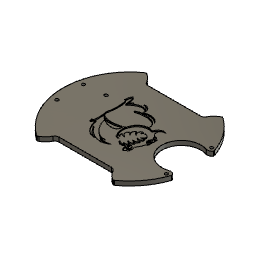
_lid.a9927ef6-e9e8-42fb-b627-377640e20614 (Autodesk Fusion 360 design; units mm, degrees)
Autodesk Fusion 360 part; units mm, degrees
sketch "reference" plane through (0, 0, 0) normal (0, 1, 0) x (1, 0, 0)
  line L0 (26.708, 42.6236) -> (27.1586, 42.6236)
  line L1 (-27.225, -55.0823) -> (17.225, -55.0823)
  line L2 (17.225, -55.0823) -> (17.225, -42.3823)
  line L3 (17.225, -42.3823) -> (-27.225, -42.3823)
  line L4 (-27.225, -42.3823) -> (-27.225, -55.0823)
  circle A0 centre (0, 0) radius 65
  line L5 (-27.225, 55.0823) -> (17.225, 55.0823)
  line L6 (17.225, 55.0823) -> (17.225, 42.3823)
  line L7 (17.225, 42.3823) -> (-27.225, 42.3823)
  line L8 (-27.225, 55.0823) -> (-27.225, 42.3823)
  circle A1 centre (0, 0) radius 67.15
  circle A2 centre (68.0978, 18.2467) radius 3
  circle A3 centre (68.0978, 18.2467) radius 1.425
  line L9 (0, 0) -> (82, 0) construction
  line L10 (0, 0) -> (-41, 71.0141) construction
  line L11 (0, 0) -> (-41, -71.0141) construction
  line L12 (87.4769, -0.0257) -> (79.614, 0.0081)
  line L13 (-39.814, 68.9437) -> (-43.7162, 75.77)
  line L14 (-39.8, -68.9518) -> (-43.7607, -75.7444)
  line L15 (0, 0) -> (70.5, 0) construction
  arc A4 (79.614, 0.0081) -> (74.6944, -3.9877) centre (79.5926, -4.9919) ccw
  arc A5 (-39.814, 68.9437) -> (-33.8938, 66.6811) centre (-35.4732, 71.4251) ccw
  arc A6 (-39.8, -68.9518) -> (-40.8007, -62.6934) centre (-44.1194, -66.4332) ccw
  spline S0 degree 5 poles (-33.8938, 66.6811) (-33.483, 66.8179) (-33.0729, 66.9532) (-32.6634, 67.087) (-32.2547, 67.2193) (-31.8466, 67.3502) knots 0.021144 0.021144 0.021144 0.021144 0.021144 0.021144 0.032444 0.032444 0.032444 0.032444 0.032444 0.032444
  line L16 (-32.0549, 67.2834) -> (-31.6382, 67.417)
  spline S1 degree 5 poles (5.0849, 74.3263) (6.6179, 74.3731) (11.2429, 74.4207) (18.7539, 74.0099) (28.746, 72.2391) (40.5731, 67.6689) (52.3904, 59.5578) (62.916, 48.5693) (72.252, 34.9305) (78.8493, 22.0782) (83.3385, 11.4171) (86.1309, 3.8631) (87.4769, -0.0257) knots 0.251095 0.251095 0.251095 0.251095 0.251095 0.251095 0.3 0.4 0.5 0.6 0.7 0.8 0.9 1 1 1 1 1 1
  line L17 (-9.3123, 73.8863) -> (19.482, 74.7663)
  spline S2 degree 5 poles (-40.8007, -62.6934) (-41.1245, -62.4061) (-41.4467, -62.1186) (-41.7673, -61.8309) (-42.0863, -61.543) (-42.4037, -61.255) knots 0.021144 0.021144 0.021144 0.021144 0.021144 0.021144 0.032444 0.032444 0.032444 0.032444 0.032444 0.032444
  line L18 (-42.2416, -61.4021) -> (-42.5658, -61.1079)
  spline S3 degree 5 poles (-66.9109, -32.7595) (-67.718, -31.4553) (-70.0717, -27.4737) (-73.4714, -20.7636) (-76.9339, -11.2248) (-78.8895, 1.3029) (-77.7737, 15.5925) (-73.5202, 30.2022) (-66.3767, 45.1068) (-58.5449, 57.2464) (-51.5568, 66.4647) (-46.4109, 72.66) (-43.7162, 75.77) knots 0.251095 0.251095 0.251095 0.251095 0.251095 0.251095 0.3 0.4 0.5 0.6 0.7 0.8 0.9 1 1 1 1 1 1
  line L19 (-59.9171, -44.0611) -> (-73.9047, -21.4578)
  arc A7 (-66.9109, -32.7595) -> (-37.25, -64.5189) centre (0, 0) ccw
  spline S4 degree 5 poles (74.6944, -3.9877) (74.6075, -4.4118) (74.5196, -4.8346) (74.4308, -5.2561) (74.341, -5.6763) (74.2503, -6.0951) knots 0.021144 0.021144 0.021144 0.021144 0.021144 0.021144 0.032444 0.032444 0.032444 0.032444 0.032444 0.032444
  line L20 (74.2965, -5.8814) -> (74.204, -6.3089)
  spline S5 degree 5 poles (61.826, -41.5668) (61.1001, -42.9178) (58.8287, -46.947) (54.7175, -53.2463) (48.1879, -61.0143) (38.3164, -68.9717) (25.3834, -75.1503) (10.6042, -78.7715) (-5.8753, -80.0373) (-20.3044, -79.3246) (-31.7817, -77.8819) (-39.7199, -76.523) (-43.7607, -75.7444) knots 0.251095 0.251095 0.251095 0.251095 0.251095 0.251095 0.3 0.4 0.5 0.6 0.7 0.8 0.9 1 1 1 1 1 1
  line L21 (68.2252, -29.657) -> (55.4268, -53.4766)
  arc A8 (61.826, -41.5668) -> (74.5, 0) centre (0, 0) ccw
  arc A9 (5.0849, 74.3263) -> (-37.25, 64.5189) centre (0, 0) ccw
  circle A10 centre (18.2467, 68.0978) radius 3
  circle A11 centre (18.2467, 68.0978) radius 1.425
  circle A12 centre (-49.851, 49.851) radius 3
  circle A13 centre (-49.851, 49.851) radius 1.425
  circle A14 centre (-68.0978, -18.2467) radius 3
  circle A15 centre (-68.0978, -18.2467) radius 1.425
  circle A16 centre (-18.2467, -68.0978) radius 3
  circle A17 centre (-18.2467, -68.0978) radius 1.425
  circle A18 centre (49.851, -49.851) radius 3
  circle A19 centre (49.851, -49.851) radius 1.425
  line L22 (0, 0) -> (55.15, 0) construction
  line L23 (0, 0) -> (55.15, 0) construction
  circle A20 centre (42.2474, -35.4497) radius 12
  circle A21 centre (42.2474, 35.4497) radius 12
  line L24 (0, 0) -> (55.15, 0) construction
  line L25 (0, 0) -> (55.15, 0) construction
  circle A22 centre (-42.2474, 35.4497) radius 12
  circle A23 centre (-42.2474, -35.4497) radius 12
  circle A24 centre (0, 0) radius 62.5
  line L26 (-5, -42.3823) -> (-5, 42.3823)
  point P0 (39, 67.55)
  point P1 (-78, 0)
  point P2 (39, -67.55)
  dimension "d9" = 12.7
  dimension "d10" = 44.45
  dimension "d53" = 12.7
  dimension "d54" = 44.45
  dimension "d63" = 130
  dimension "d76" = 134.3
  dimension "d123" = 78
  dimension "d127" = 5
  dimension "d128" = 5
  dimension "d129" = 5
  dimension "d132" = 149
  dimension "d136" = 360
  dimension "d204" = 55.15
  dimension "d206" = 55.15
  dimension "d207" = 24
  dimension "d208" = 24
  dimension "d210" = 55.15
  dimension "d212" = 55.15
  dimension "d213" = 24
  dimension "d214" = 24
  dimension "d227" = 125
  dimension "d232" = 84.7646
  constraint perpendicular L1 L2
  constraint perpendicular L2 L3
  constraint coincident A0.centre A1.centre
  constraint perpendicular L5 L6
  constraint perpendicular L6 L7
  constraint horizontal L9
  constraint horizontal L15
  constraint tangent A4 S4
  constraint tangent L12 A4
  constraint tangent A5 S0
  constraint tangent L13 A5
  constraint tangent A6 S2
  constraint tangent L14 A6
  constraint coincident S0.end A7
  constraint midpoint S0.end L16
  constraint coincident S1.start A7
  constraint midpoint S1.start L17
  constraint coincident L10 A9.end
  constraint coincident S2.end A7
  constraint midpoint S2.end L18
  constraint midpoint S3.start L19
  constraint coincident L11 A7.end
  constraint concentric A7 A8
  constraint coincident S4.end A8
  constraint midpoint S4.end L20
  constraint midpoint S5.start L21
  constraint coincident L9 A8.end
  constraint concentric A8 A9
  constraint horizontal L22
  constraint horizontal L23
  constraint horizontal L24
  constraint horizontal L25
  constraint midpoint L3 L26.start
  constraint midpoint L7 L26.end
  constraint perpendicular L7 L26
  measures "d9" distance of L1.end L2.end
  measures "d10" distance of L2.end L3.end
  measures "d53" distance of L5.end L6.end
  measures "d54" distance of L6.end L7.end
  measures "d63" diameter of A0
  measures "d76" diameter of A1
  measures "d123" distance of A0.centre P0
  measures "d127" radius of A4
  measures "d128" radius of A5
  measures "d129" radius of A6
  measures "d132" diameter of A7
  measures "d204" distance of A0.centre A20.centre
  measures "d206" distance of A0.centre A21.centre
  measures "d207" diameter of A20
  measures "d208" diameter of A21
  measures "d210" distance of A0.centre A23.centre
  measures "d212" distance of A0.centre A22.centre
  measures "d213" diameter of A22
  measures "d214" diameter of A23
  measures "d227" diameter of A24
  measures "d232" distance of L26.start L26.end
sketch "Sketch6" plane through (0, 0, 0) normal (0, 1, 0) x (1, 0, 0)
  line L0 (-18.5, 40.9998) -> (8.5, 40.9998)
  line L1 (24.1077, -40.9998) -> (-24.1077, -40.9998)
  line L2 (-18.5, 40.9998) -> (8.5, 40.9998)
  line L3 (-5, 40.9998) -> (-24.1077, 40.9998)
  line L4 (-5, 40.9998) -> (24.173, 40.9998)
  arc A0 (33.8961, 49.6132) -> (27.7096, 43.1311) centre (42.2474, 35.4497) ccw
  arc A1 (-27.6472, 43.1364) -> (-33.8408, 49.6476) centre (-42.2474, 35.4497) ccw
  arc A2 (-33.8408, -49.6476) -> (-27.6472, -43.1364) centre (-42.2474, -35.4497) ccw
  arc A3 (27.6472, -43.1364) -> (33.8408, -49.6476) centre (42.2474, -35.4497) ccw
  arc A4 (-24.1077, -40.9998) -> (-27.6472, -43.1364) centre (-24.1077, -44.9998) ccw
  arc A5 (27.6472, -43.1364) -> (24.1077, -40.9998) centre (24.1077, -44.9998) ccw
  arc A6 (24.173, 40.9998) -> (27.7096, 43.1311) centre (24.173, 44.9998) ccw
  arc A7 (-27.6472, 43.1364) -> (-24.1077, 40.9998) centre (-24.1077, 44.9998) ccw
  arc A8 (-33.8408, 49.6476) -> (-35.0849, 50.1261) centre (-35.8787, 46.2057) ccw
  arc A9 (35.1381, 50.0889) -> (33.8961, 49.6132) centre (35.9277, 46.1676) ccw
  arc A10 (-35.5399, -50.1913) -> (-33.8408, -49.6476) centre (-35.8787, -46.2057) ccw
  arc A11 (33.8408, -49.6476) -> (35.5399, -50.1913) centre (35.8787, -46.2057) ccw
  arc A12 (58.1788, -18.9422) -> (53.3811, -17.0548) centre (54.6603, -20.8448) ccw
  arc A13 (53.3811, 17.0548) -> (58.1788, 18.9422) centre (54.6603, 20.8448) ccw
  line L5 (25.625, -0.0248) -> (25.625, 0.0248)
  line L6 (-24.375, 0.0248) -> (-24.375, 0)
  line L7 (0, 0) -> (-24.375, 0) construction
  line L8 (-62.5, 0) -> (-63.5, 0) construction
  circle A14 centre (54.6603, 20.8448) radius 1.425
  circle A15 centre (54.6603, -20.8448) radius 1.425
  circle A16 centre (-54.8646, 12.1784) radius 1.425
  circle A17 centre (-54.8646, -12.1784) radius 1.425
  arc A18 (53.3811, 17.0548) -> (53.3811, -17.0548) centre (47.625, 0) ccw
  spline S0 degree 3 poles (23.6109, 1.2589) (23.5474, 1.4494) (23.3887, 1.7272) (23.2458, 1.8701) knots 0 0 0 0 1 1 1 1
  spline S1 degree 3 poles (23.2458, 1.8701) (22.6664, 2.4654) (21.9123, 2.2591) (21.0868, 1.2669) knots 0 0 0 0 1 1 1 1
  line L9 (21.0868, 1.2669) -> (20.8646, 1.0049)
  line L10 (20.8646, 1.0049) -> (20.6503, 1.2034)
  spline S2 degree 3 poles (20.6503, 1.2034) (20.5312, 1.3066) (20.3407, 1.4574) (20.2296, 1.5288) knots 0 0 0 0 1 1 1 1
  spline S3 degree 3 poles (20.2296, 1.5288) (20.0311, 1.6479) (19.6263, 2.1956) (19.6898, 2.2511) knots 0 0 0 0 1 1 1 1
  spline S4 degree 3 poles (19.6898, 2.2511) (19.7057, 2.2591) (19.8803, 2.3543) (20.0788, 2.4496) knots 0 0 0 0 1 1 1 1
  spline S5 degree 3 poles (20.0788, 2.4496) (20.4756, 2.648) (21.4281, 3.2671) (21.4281, 3.3306) knots 0 0 0 0 1 1 1 1
  spline S6 degree 3 poles (21.4281, 3.3306) (21.4281, 3.3544) (21.2614, 3.3624) (21.0551, 3.3465) knots 0 0 0 0 1 1 1 1
  spline S7 degree 3 poles (21.0551, 3.3465) (20.5391, 3.3068) (19.6739, 3.5211) (19.1183, 3.8148) knots 0 0 0 0 1 1 1 1
  spline S8 degree 3 poles (19.1183, 3.8148) (18.269, 4.2752) (17.5149, 5.2436) (17.253, 6.2278) knots 0 0 0 0 1 1 1 1
  spline S9 degree 3 poles (17.253, 6.2278) (17.1101, 6.7596) (17.1181, 7.6327) (17.2609, 8.2122) knots 0 0 0 0 1 1 1 1
  spline S10 degree 3 poles (17.2609, 8.2122) (17.6419, 9.6727) (18.8961, 10.8395) (20.428, 11.1649) knots 0 0 0 0 1 1 1 1
  spline S11 degree 3 poles (20.428, 11.1649) (20.7614, 11.2364) (21.1662, 11.2602) (21.4281, 11.2364) knots 0 0 0 0 1 1 1 1
  line L11 (21.4281, 11.2364) -> (21.8647, 11.1887)
  line L12 (21.8647, 11.1887) -> (21.571, 11.3475)
  spline S12 degree 3 poles (21.571, 11.3475) (20.6503, 11.8396) (19.0945, 11.8793) (17.9674, 11.4348) knots 0 0 0 0 1 1 1 1
  spline S13 degree 3 poles (17.9674, 11.4348) (16.4116, 10.8316) (15.2289, 9.7203) (14.4908, 8.1804) knots 0 0 0 0 1 1 1 1
  spline S14 degree 3 poles (14.4908, 8.1804) (14.3399, 7.855) (14.1733, 7.4105) (14.1177, 7.1803) knots 0 0 0 0 1 1 1 1
  line L13 (14.1177, 7.1803) -> (14.0224, 6.7596)
  line L14 (14.0224, 6.7596) -> (13.5779, 6.9104)
  spline S15 degree 3 poles (13.5779, 6.9104) (12.1492, 7.4026) (9.9743, 7.5613) (8.4424, 7.2756) knots 0 0 0 0 1 1 1 1
  spline S16 degree 3 poles (8.4424, 7.2756) (1.8146, 6.0532) (-2.5511, -1.1223) (-1.0191, -8.2581) knots 0 0 0 0 1 1 1 1
  spline S17 degree 3 poles (-1.0191, -8.2581) (-0.7334, -9.5996) (-0.1619, -11.1394) (0.6398, -12.7666) knots 0 0 0 0 1 1 1 1
  spline S18 degree 3 poles (0.6398, -12.7666) (1.1478, -13.7826) (2.1638, -14.5288) (3.1401, -14.5923) knots 0 0 0 0 1 1 1 1
  spline S19 degree 3 poles (3.1401, -14.5923) (3.6402, -14.624) (4.1244, -14.5208) (4.2672, -14.3462) knots 0 0 0 0 1 1 1 1
  spline S20 degree 3 poles (4.2672, -14.3462) (4.3307, -14.2748) (4.2593, -14.2509) (4.0132, -14.243) knots 0 0 0 0 1 1 1 1
  spline S21 degree 3 poles (4.0132, -14.243) (2.7591, -14.2113) (1.5129, -12.8936) (1.3224, -11.4173) knots 0 0 0 0 1 1 1 1
  spline S22 degree 3 poles (1.3224, -11.4173) (1.2907, -11.1871) (1.2986, -11.0363) (1.3462, -11.0363) knots 0 0 0 0 1 1 1 1
  spline S23 degree 3 poles (1.3462, -11.0363) (1.3939, -11.0363) (1.4256, -11.0839) (1.4256, -11.1474) knots 0 0 0 0 1 1 1 1
  spline S24 degree 3 poles (1.4256, -11.1474) (1.4256, -11.2109) (1.6082, -11.4569) (1.8225, -11.703) knots 0 0 0 0 1 1 1 1
  spline S25 degree 3 poles (1.8225, -11.703) (2.2194, -12.1316) (2.5686, -12.3221) (3.156, -12.4174) knots 0 0 0 0 1 1 1 1
  spline S26 degree 3 poles (3.156, -12.4174) (3.4259, -12.465) (3.5132, -12.3459) (3.2592, -12.2666) knots 0 0 0 0 1 1 1 1
  spline S27 degree 3 poles (3.2592, -12.2666) (3.0211, -12.1951) (2.4654, -11.5443) (2.2987, -11.1553) knots 0 0 0 0 1 1 1 1
  spline S28 degree 3 poles (2.2987, -11.1553) (2.0765, -10.6473) (1.9654, -9.8933) (2.0289, -9.4011) knots 0 0 0 0 1 1 1 1
  line L15 (2.0289, -9.4011) -> (2.0765, -8.9646)
  line L16 (2.0765, -8.9646) -> (2.3464, -9.2821)
  spline S29 degree 3 poles (2.3464, -9.2821) (2.9972, -10.0441) (4.1482, -10.56) (5.188, -10.56) knots 0 0 0 0 1 1 1 1
  spline S30 degree 3 poles (5.188, -10.56) (5.8468, -10.56) (6.1246, -10.4489) (5.6563, -10.3774) knots 0 0 0 0 1 1 1 1
  spline S31 degree 3 poles (5.6563, -10.3774) (4.8546, -10.2504) (3.7513, -9.3932) (3.3386, -8.5915) knots 0 0 0 0 1 1 1 1
  spline S32 degree 3 poles (3.3386, -8.5915) (2.5845, -7.1231) (2.9972, -5.5356) (4.299, -4.8926) knots 0 0 0 0 1 1 1 1
  line L17 (4.299, -4.8926) -> (4.7038, -4.6863)
  line L18 (4.7038, -4.6863) -> (4.9578, -5.0673)
  spline S33 degree 3 poles (4.9578, -5.0673) (5.2991, -5.5673) (5.8468, -6.0594) (6.3389, -6.3055) knots 0 0 0 0 1 1 1 1
  spline S34 degree 3 poles (6.3389, -6.3055) (6.5612, -6.4166) (6.7596, -6.5119) (6.7914, -6.5119) knots 0 0 0 0 1 1 1 1
  spline S35 degree 3 poles (6.7914, -6.5119) (6.8231, -6.5119) (6.6803, -6.3373) (6.4818, -6.1229) knots 0 0 0 0 1 1 1 1
  spline S36 degree 3 poles (6.4818, -6.1229) (5.1483, -4.7021) (5.2674, -2.4082) (6.7358, -1.2969) knots 0 0 0 0 1 1 1 1
  spline S37 degree 3 poles (6.7358, -1.2969) (6.9184, -1.1541) (7.1168, -1.035) (7.1803, -1.035) knots 0 0 0 0 1 1 1 1
  spline S38 degree 3 poles (7.1803, -1.035) (7.2359, -1.035) (7.3232, -1.2017) (7.3708, -1.4001) knots 0 0 0 0 1 1 1 1
  spline S39 degree 3 poles (7.3708, -1.4001) (7.6566, -2.5352) (8.6964, -3.6226) (9.7203, -3.8608) knots 0 0 0 0 1 1 1 1
  spline S40 degree 3 poles (9.7203, -3.8608) (9.9584, -3.9163) (9.9584, -3.9084) (9.6251, -3.6226) knots 0 0 0 0 1 1 1 1
  spline S41 degree 3 poles (9.6251, -3.6226) (8.5932, -2.7257) (8.2122, -1.1541) (8.744, 0.0048) knots 0 0 0 0 1 1 1 1
  spline S42 degree 3 poles (8.744, 0.0048) (9.1726, 0.9335) (9.7918, 1.3462) (10.7601, 1.3462) knots 0 0 0 0 1 1 1 1
  spline S43 degree 3 poles (10.7601, 1.3462) (11.0776, 1.3462) (11.3634, 1.3066) (11.3872, 1.2669) knots 0 0 0 0 1 1 1 1
  spline S44 degree 3 poles (11.3872, 1.2669) (11.411, 1.2192) (11.3634, 1.0764) (11.2681, 0.9494) knots 0 0 0 0 1 1 1 1
  spline S45 degree 3 poles (11.2681, 0.9494) (11.0538, 0.6477) (10.7919, -0.0904) (10.7919, -0.3762) knots 0 0 0 0 1 1 1 1
  spline S46 degree 3 poles (10.7919, -0.3762) (10.7998, -0.5984) (10.7998, -0.5984) (10.9506, -0.3127) knots 0 0 0 0 1 1 1 1
  spline S47 degree 3 poles (10.9506, -0.3127) (11.284, 0.3144) (12.1413, 0.87) (13.0541, 1.0367) knots 0 0 0 0 1 1 1 1
  spline S48 degree 3 poles (13.0541, 1.0367) (13.9272, 1.1954) (14.9908, 0.8779) (15.602, 0.2667) knots 0 0 0 0 1 1 1 1
  spline S49 degree 3 poles (15.602, 0.2667) (16.8641, -1.0033) (16.2449, -3.0353) (14.4034, -3.6544) knots 0 0 0 0 1 1 1 1
  line L19 (14.4034, -3.6544) -> (13.9272, -3.8131)
  line L20 (13.9272, -3.8131) -> (14.5622, -3.7893)
  spline S50 degree 3 poles (14.5622, -3.7893) (15.2448, -3.7496) (15.8878, -3.5512) (16.3958, -3.2099) knots 0 0 0 0 1 1 1 1
  spline S51 degree 3 poles (16.3958, -3.2099) (16.7371, -2.9797) (16.7767, -3.0114) (16.8958, -3.575) knots 0 0 0 0 1 1 1 1
  spline S52 degree 3 poles (16.8958, -3.575) (17.0466, -4.2656) (16.6974, -5.1228) (16.0862, -5.5673) knots 0 0 0 0 1 1 1 1
  spline S53 degree 3 poles (16.0862, -5.5673) (15.1654, -6.2341) (13.9986, -6.3452) (12.9985, -5.8451) knots 0 0 0 0 1 1 1 1
  spline S54 degree 3 poles (12.9985, -5.8451) (12.7842, -5.7499) (12.6175, -5.6864) (12.6175, -5.7261) knots 0 0 0 0 1 1 1 1
  spline S55 degree 3 poles (12.6175, -5.7261) (12.6175, -5.8848) (13.5383, -6.5992) (13.951, -6.7579) knots 0 0 0 0 1 1 1 1
  spline S56 degree 3 poles (13.951, -6.7579) (14.4828, -6.9564) (15.3718, -7.0358) (15.8719, -6.9167) knots 0 0 0 0 1 1 1 1
  spline S57 degree 3 poles (15.8719, -6.9167) (16.0624, -6.877) (16.237, -6.8532) (16.2529, -6.8611) knots 0 0 0 0 1 1 1 1
  spline S58 degree 3 poles (16.2529, -6.8611) (16.3561, -6.9643) (16.3481, -7.5199) (16.2291, -7.9009) knots 0 0 0 0 1 1 1 1
  spline S59 degree 3 poles (16.2291, -7.9009) (15.8163, -9.3297) (13.7605, -10.0441) (12.3238, -9.2503) knots 0 0 0 0 1 1 1 1
  spline S60 degree 3 poles (12.3238, -9.2503) (12.1333, -9.1471) (11.9825, -9.0916) (11.9825, -9.1233) knots 0 0 0 0 1 1 1 1
  spline S61 degree 3 poles (11.9825, -9.1233) (11.9825, -9.2741) (12.8159, -9.9488) (13.2366, -10.1473) knots 0 0 0 0 1 1 1 1
  spline S62 degree 3 poles (13.2366, -10.1473) (13.6414, -10.3378) (13.7843, -10.3616) (14.5384, -10.3616) knots 0 0 0 0 1 1 1 1
  spline S63 degree 3 poles (14.5384, -10.3616) (15.1734, -10.3616) (15.3956, -10.3854) (15.3956, -10.4648) knots 0 0 0 0 1 1 1 1
  spline S64 degree 3 poles (15.3956, -10.4648) (15.3956, -10.6949) (15.0146, -11.3458) (14.6733, -11.6871) knots 0 0 0 0 1 1 1 1
  spline S65 degree 3 poles (14.6733, -11.6871) (13.6732, -12.6873) (12.0619, -12.9095) (10.6887, -12.2269) knots 0 0 0 0 1 1 1 1
  line L21 (10.6887, -12.2269) -> (10.2362, -11.9967)
  line L22 (10.2362, -11.9967) -> (10.395, -12.2269)
  spline S66 degree 3 poles (10.395, -12.2269) (10.9744, -13.0365) (12.1333, -13.6001) (13.2684, -13.608) knots 0 0 0 0 1 1 1 1
  spline S67 degree 3 poles (13.2684, -13.608) (13.6097, -13.6159) (13.8875, -13.6239) (13.8875, -13.6398) knots 0 0 0 0 1 1 1 1
  spline S68 degree 3 poles (13.8875, -13.6398) (13.8875, -13.7826) (13.4668, -14.4018) (13.1414, -14.7272) knots 0 0 0 0 1 1 1 1
  spline S69 degree 3 poles (13.1414, -14.7272) (12.3953, -15.4813) (11.3237, -15.8305) (10.1966, -15.7114) knots 0 0 0 0 1 1 1 1
  spline S70 degree 3 poles (10.1966, -15.7114) (9.9346, -15.6797) (9.7124, -15.6638) (9.6965, -15.6797) knots 0 0 0 0 1 1 1 1
  spline S71 degree 3 poles (9.6965, -15.6797) (9.6092, -15.767) (10.903, -16.2909) (11.2919, -16.3306) knots 0 0 0 0 1 1 1 1
  spline S72 degree 3 poles (11.2919, -16.3306) (11.7364, -16.3782) (11.7444, -16.3782) (11.6094, -16.529) knots 0 0 0 0 1 1 1 1
  spline S73 degree 3 poles (11.6094, -16.529) (11.538, -16.6084) (11.2522, -16.7909) (10.9744, -16.9259) knots 0 0 0 0 1 1 1 1
  spline S74 degree 3 poles (10.9744, -16.9259) (9.6647, -17.5688) (7.9502, -17.1719) (6.9104, -15.9893) knots 0 0 0 0 1 1 1 1
  spline S75 degree 3 poles (6.9104, -15.9893) (6.5215, -15.5448) (6.5215, -15.6559) (6.9025, -16.4734) knots 0 0 0 0 1 1 1 1
  spline S76 degree 3 poles (6.9025, -16.4734) (7.3232, -17.3863) (8.1884, -18.1165) (9.2203, -18.4261) knots 0 0 0 0 1 1 1 1
  spline S77 degree 3 poles (9.2203, -18.4261) (10.0537, -18.6801) (11.1094, -18.6245) (11.8634, -18.2753) knots 0 0 0 0 1 1 1 1
  spline S78 degree 3 poles (11.8634, -18.2753) (12.173, -18.1324) (12.6889, -17.9498) (13.0144, -17.8625) knots 0 0 0 0 1 1 1 1
  spline S79 degree 3 poles (13.0144, -17.8625) (13.3398, -17.7831) (13.6811, -17.6879) (13.7684, -17.6641) knots 0 0 0 0 1 1 1 1
  spline S80 degree 3 poles (13.7684, -17.6641) (13.9193, -17.6164) (13.9272, -17.6641) (13.951, -18.3149) knots 0 0 0 0 1 1 1 1
  spline S81 degree 3 poles (13.951, -18.3149) (14.0145, -19.9342) (14.5384, -21.3153) (15.2607, -21.7519) knots 0 0 0 0 1 1 1 1
  spline S82 degree 3 poles (15.2607, -21.7519) (15.5623, -21.9424) (16.1021, -21.9583) (16.4196, -21.7916) knots 0 0 0 0 1 1 1 1
  spline S83 degree 3 poles (16.4196, -21.7916) (16.7053, -21.6487) (17.1736, -21.101) (17.3641, -20.7121) knots 0 0 0 0 1 1 1 1
  spline S84 degree 3 poles (17.3641, -20.7121) (17.4991, -20.4184) (17.4991, -20.4184) (17.9039, -20.4581) knots 0 0 0 0 1 1 1 1
  spline S85 degree 3 poles (17.9039, -20.4581) (18.6024, -20.5295) (18.9675, -20.212) (19.2374, -19.2992) knots 0 0 0 0 1 1 1 1
  spline S86 degree 3 poles (19.2374, -19.2992) (19.5549, -18.2197) (19.4438, -16.7274) (18.9278, -15.1876) knots 0 0 0 0 1 1 1 1
  line L23 (18.9278, -15.1876) -> (18.65, -14.3541)
  line L24 (18.65, -14.3541) -> (18.9596, -13.9811)
  spline S87 degree 3 poles (18.9596, -13.9811) (19.8486, -12.9174) (20.7455, -11.2744) (21.2218, -9.8456) knots 0 0 0 0 1 1 1 1
  spline S88 degree 3 poles (21.2218, -9.8456) (21.4996, -9.0122) (21.825, -7.5834) (21.825, -7.1945) knots 0 0 0 0 1 1 1 1
  spline S89 degree 3 poles (21.825, -7.1945) (21.825, -6.9961) (21.8488, -6.9881) (22.2219, -6.9881) knots 0 0 0 0 1 1 1 1
  spline S90 degree 3 poles (22.2219, -6.9881) (22.7696, -6.9881) (23.0394, -6.8294) (23.2617, -6.3769) knots 0 0 0 0 1 1 1 1
  spline S91 degree 3 poles (23.2617, -6.3769) (23.4284, -6.0356) (23.4522, -5.8928) (23.4522, -5.0038) knots 0 0 0 0 1 1 1 1
  spline S92 degree 3 poles (23.4522, -5.0038) (23.4443, -4.2497) (23.4046, -3.8608) (23.2776, -3.3845) knots 0 0 0 0 1 1 1 1
  spline S93 degree 3 poles (23.2776, -3.3845) (23.1188, -2.8051) (23.1109, -2.7336) (23.222, -2.5193) knots 0 0 0 0 1 1 1 1
  spline S94 degree 3 poles (23.222, -2.5193) (23.2934, -2.3923) (23.4363, -1.9478) (23.5395, -1.5351) knots 0 0 0 0 1 1 1 1
  spline S95 degree 3 poles (23.5395, -1.5351) (23.7618, -0.6619) (23.7935, 0.6716) (23.6109, 1.2589) knots 0 0 0 0 1 1 1 1
  spline S96 degree 3 poles (23.3728, -1.6303) (23.0871, -2.7495) (22.2139, -4.0116) (21.3884, -4.4958) knots 0 0 0 0 1 1 1 1
  spline S97 degree 3 poles (21.3884, -4.4958) (20.9836, -4.7339) (20.428, -4.8133) (20.1581, -4.6704) knots 0 0 0 0 1 1 1 1
  spline S98 degree 3 poles (20.1581, -4.6704) (19.6422, -4.3926) (19.4438, -3.6941) (19.6343, -2.7733) knots 0 0 0 0 1 1 1 1
  spline S99 degree 3 poles (19.6343, -2.7733) (19.9438, -1.3128) (21.1027, 0.1953) (22.1584, 0.4731) knots 0 0 0 0 1 1 1 1
  spline S100 degree 3 poles (22.1584, 0.4731) (23.1823, 0.7509) (23.7379, -0.2095) (23.3728, -1.6303) knots 0 0 0 0 1 1 1 1
  spline S101 degree 3 poles (17.4038, -17.7196) (17.1974, -18.0689) (16.7926, -18.1165) (16.4513, -17.8308) knots 0 0 0 0 1 1 1 1
  spline S102 degree 3 poles (16.4513, -17.8308) (15.9354, -17.4021) (15.4988, -16.148) (15.5861, -15.3622) knots 0 0 0 0 1 1 1 1
  spline S103 degree 3 poles (15.5861, -15.3622) (15.6179, -15.0526) (15.6099, -14.9971) (15.5385, -15.1161) knots 0 0 0 0 1 1 1 1
  spline S104 degree 3 poles (15.5385, -15.1161) (15.4909, -15.2034) (15.4671, -15.5527) (15.4909, -15.9893) knots 0 0 0 0 1 1 1 1
  spline S105 degree 3 poles (15.4909, -15.9893) (15.5147, -16.5925) (15.5623, -16.7989) (15.7607, -17.2275) knots 0 0 0 0 1 1 1 1
  spline S106 degree 3 poles (15.7607, -17.2275) (15.8957, -17.5133) (16.1259, -17.8625) (16.2767, -18.0054) knots 0 0 0 0 1 1 1 1
  line L25 (16.2767, -18.0054) -> (16.5386, -18.2594)
  line L26 (16.5386, -18.2594) -> (16.3243, -18.4737)
  spline S107 degree 3 poles (16.3243, -18.4737) (16.0862, -18.7118) (15.6576, -18.7674) (15.4353, -18.5769) knots 0 0 0 0 1 1 1 1
  spline S108 degree 3 poles (15.4353, -18.5769) (15.0305, -18.2356) (14.7844, -17.1958) (14.9194, -16.3464) knots 0 0 0 0 1 1 1 1
  spline S109 degree 3 poles (14.9194, -16.3464) (15.0226, -15.6479) (15.221, -15.2273) (15.6734, -14.751) knots 0 0 0 0 1 1 1 1
  spline S110 degree 3 poles (15.6734, -14.751) (16.1417, -14.243) (16.3402, -14.243) (16.8164, -14.751) knots 0 0 0 0 1 1 1 1
  spline S111 degree 3 poles (16.8164, -14.751) (17.1657, -15.1003) (17.4514, -15.7273) (17.5705, -16.3544) knots 0 0 0 0 1 1 1 1
  spline S112 degree 3 poles (17.5705, -16.3544) (17.6419, -16.7433) (17.5546, -17.4656) (17.4038, -17.7196) knots 0 0 0 0 1 1 1 1
  spline S113 degree 3 poles (21.7139, -0.8207) (21.2059, 0.2826) (19.6263, -1.8367) (19.7851, -3.4004) knots 0 0 0 0 1 1 1 1
  spline S114 degree 3 poles (19.7851, -3.4004) (19.9597, -5.0673) (21.6742, -3.5512) (21.7933, -1.6303) knots 0 0 0 0 1 1 1 1
  spline S115 degree 3 poles (21.7933, -1.6303) (21.8171, -1.2493) (21.7933, -0.9953) (21.7139, -0.8207) knots 0 0 0 0 1 1 1 1
  spline S116 degree 3 poles (9.5695, 10.3712) (9.4187, 10.9824) (8.8789, 12.0381) (8.4344, 12.5778) knots 0 0 0 0 1 1 1 1
  spline S117 degree 3 poles (8.4344, 12.5778) (7.0454, 14.2764) (4.5609, 15.4194) (1.3463, 15.8401) knots 0 0 0 0 1 1 1 1
  spline S118 degree 3 poles (1.3463, 15.8401) (0.0286, 16.0148) (-2.5272, 16.0148) (-4.0116, 15.8401) knots 0 0 0 0 1 1 1 1
  spline S119 degree 3 poles (-4.0116, 15.8401) (-5.9324, 15.6099) (-8.8217, 14.9591) (-10.0441, 14.4749) knots 0 0 0 0 1 1 1 1
  spline S120 degree 3 poles (-10.0441, 14.4749) (-10.2187, 14.4114) (-10.3219, 14.3876) (-10.2743, 14.4431) knots 0 0 0 0 1 1 1 1
  spline S121 degree 3 poles (-10.2743, 14.4431) (-10.1314, 14.586) (-7.7263, 15.5941) (-6.6706, 15.9513) knots 0 0 0 0 1 1 1 1
  spline S122 degree 3 poles (-6.6706, 15.9513) (-0.3841, 18.0626) (5.3309, 17.6023) (7.9582, 14.7606) knots 0 0 0 0 1 1 1 1
  spline S123 degree 3 poles (7.9582, 14.7606) (8.2043, 14.4908) (8.4106, 14.3003) (8.4106, 14.332) knots 0 0 0 0 1 1 1 1
  spline S124 degree 3 poles (8.4106, 14.332) (8.4106, 14.3558) (8.2995, 14.6019) (8.1566, 14.8718) knots 0 0 0 0 1 1 1 1
  spline S125 degree 3 poles (8.1566, 14.8718) (7.9899, 15.1813) (7.6486, 15.6099) (7.1883, 16.0703) knots 0 0 0 0 1 1 1 1
  spline S126 degree 3 poles (7.1883, 16.0703) (6.3945, 16.8641) (5.5849, 17.3483) (4.4339, 17.7213) knots 0 0 0 0 1 1 1 1
  spline S127 degree 3 poles (4.4339, 17.7213) (2.9099, 18.2214) (0.4573, 18.3563) (-1.5509, 18.0626) knots 0 0 0 0 1 1 1 1
  spline S128 degree 3 poles (-1.5509, 18.0626) (-2.3844, 17.9356) (-4.4084, 17.4832) (-4.7736, 17.3403) knots 0 0 0 0 1 1 1 1
  spline S129 degree 3 poles (-4.7736, 17.3403) (-4.8926, 17.2927) (-4.9006, 17.3324) (-4.8291, 17.6737) knots 0 0 0 0 1 1 1 1
  spline S130 degree 3 poles (-4.8291, 17.6737) (-4.6942, 18.3166) (-4.718, 19.9756) (-4.8688, 20.555) knots 0 0 0 0 1 1 1 1
  spline S131 degree 3 poles (-4.8688, 20.555) (-5.3212, 22.3013) (-6.4642, 23.4284) (-8.1152, 23.7776) knots 0 0 0 0 1 1 1 1
  spline S132 degree 3 poles (-8.1152, 23.7776) (-8.7582, 23.9205) (-10.3616, 23.8888) (-10.7188, 23.7379) knots 0 0 0 0 1 1 1 1
  spline S133 degree 3 poles (-10.7188, 23.7379) (-10.9093, 23.6506) (-10.9093, 23.6506) (-10.6791, 23.6903) knots 0 0 0 0 1 1 1 1
  spline S134 degree 3 poles (-10.6791, 23.6903) (-10.2346, 23.7697) (-9.2741, 23.5792) (-8.6788, 23.2934) knots 0 0 0 0 1 1 1 1
  spline S135 degree 3 poles (-8.6788, 23.2934) (-7.5517, 22.7696) (-6.6309, 21.5789) (-6.3214, 20.2772) knots 0 0 0 0 1 1 1 1
  spline S136 degree 3 poles (-6.3214, 20.2772) (-6.2658, 20.0549) (-6.2737, 20.0549) (-6.6865, 20.4439) knots 0 0 0 0 1 1 1 1
  spline S137 degree 3 poles (-6.6865, 20.4439) (-7.2262, 20.9519) (-7.6708, 21.2138) (-8.4169, 21.4361) knots 0 0 0 0 1 1 1 1
  spline S138 degree 3 poles (-8.4169, 21.4361) (-9.1789, 21.6663) (-10.4489, 21.6821) (-11.4331, 21.4758) knots 0 0 0 0 1 1 1 1
  spline S139 degree 3 poles (-11.4331, 21.4758) (-13.9334, 20.9439) (-16.7433, 19.2453) (-19.0214, 16.8879) knots 0 0 0 0 1 1 1 1
  line L27 (-19.0214, 16.8879) -> (-19.7437, 16.1418)
  line L28 (-19.7437, 16.1418) -> (-19.831, 17.5864)
  spline S140 degree 3 poles (-19.831, 17.5864) (-20.0136, 20.4121) (-20.2914, 22.0869) (-20.847, 23.8094) knots 0 0 0 0 1 1 1 1
  spline S141 degree 3 poles (-20.847, 23.8094) (-20.8708, 23.8729) (-20.8311, 23.8411) (-20.7676, 23.73) knots 0 0 0 0 1 1 1 1
  spline S142 degree 3 poles (-20.7676, 23.73) (-20.3311, 23.0236) (-19.8231, 20.4756) (-19.6246, 17.9833) knots 0 0 0 0 1 1 1 1
  line L29 (-19.6246, 17.9833) -> (-19.5691, 17.2689)
  line L30 (-19.5691, 17.2689) -> (-19.0531, 17.9833)
  spline S143 degree 3 poles (-19.0531, 17.9833) (-18.4419, 18.8246) (-17.7911, 19.5946) (-17.1243, 20.2534) knots 0 0 0 0 1 1 1 1
  spline S144 degree 3 poles (-17.1243, 20.2534) (-16.7751, 20.5947) (-16.7116, 20.682) (-16.91, 20.5471) knots 0 0 0 0 1 1 1 1
  spline S145 degree 3 poles (-16.91, 20.5471) (-17.0608, 20.4439) (-17.6641, 19.8883) (-18.2356, 19.3088) knots 0 0 0 0 1 1 1 1
  spline S146 degree 3 poles (-18.2356, 19.3088) (-18.815, 18.7294) (-19.2912, 18.2849) (-19.2912, 18.3166) knots 0 0 0 0 1 1 1 1
  spline S147 degree 3 poles (-19.2912, 18.3166) (-19.2912, 18.4913) (-19.5453, 20.2772) (-19.6484, 20.8725) knots 0 0 0 0 1 1 1 1
  spline S148 degree 3 poles (-19.6484, 20.8725) (-19.9183, 22.3251) (-20.4263, 23.73) (-20.7835, 23.984) knots 0 0 0 0 1 1 1 1
  spline S149 degree 3 poles (-20.7835, 23.984) (-20.8708, 24.0396) (-20.9899, 24.1983) (-21.0613, 24.3253) knots 0 0 0 0 1 1 1 1
  spline S150 degree 3 poles (-21.0613, 24.3253) (-21.2518, 24.7063) (-21.5931, 25) (-21.8233, 25) knots 0 0 0 0 1 1 1 1
  spline S151 degree 3 poles (-21.8233, 25) (-22.0694, 25) (-22.4504, 24.6428) (-22.6647, 24.2063) knots 0 0 0 0 1 1 1 1
  spline S152 degree 3 poles (-22.6647, 24.2063) (-23.0457, 23.4522) (-23.5219, 21.6504) (-23.7363, 20.1184) knots 0 0 0 0 1 1 1 1
  spline S153 degree 3 poles (-23.7363, 20.1184) (-23.7839, 19.7692) (-23.8394, 19.3723) (-23.8712, 19.2453) knots 0 0 0 0 1 1 1 1
  line L31 (-23.8712, 19.2453) -> (-23.9109, 19.0072)
  line L32 (-23.9109, 19.0072) -> (-23.6807, 19.2215)
  spline S154 degree 3 poles (-23.6807, 19.2215) (-23.1092, 19.7613) (-22.6171, 19.2929) (-22.1884, 17.8007) knots 0 0 0 0 1 1 1 1
  spline S155 degree 3 poles (-22.1884, 17.8007) (-21.1486, 14.2288) (-21.228, 6.585) (-22.3472, 2.14) knots 0 0 0 0 1 1 1 1
  spline S156 degree 3 poles (-22.3472, 2.14) (-22.5298, 1.4256) (-22.5298, 1.3621) (-22.4186, 0.8462) knots 0 0 0 0 1 1 1 1
  spline S157 degree 3 poles (-22.4186, 0.8462) (-22.2599, 0.0921) (-21.9424, -2.3606) (-21.8233, -3.6941) knots 0 0 0 0 1 1 1 1
  spline S158 degree 3 poles (-21.8233, -3.6941) (-21.6963, -5.1466) (-21.6963, -8.4883) (-21.8154, -9.4488) knots 0 0 0 0 1 1 1 1
  spline S159 degree 3 poles (-21.8154, -9.4488) (-21.9503, -10.4806) (-22.2123, -11.4014) (-22.4424, -11.6792) knots 0 0 0 0 1 1 1 1
  spline S160 degree 3 poles (-22.4424, -11.6792) (-22.8076, -12.1078) (-23.2441, -11.9253) (-23.6251, -11.1791) knots 0 0 0 0 1 1 1 1
  spline S161 degree 3 poles (-23.6251, -11.1791) (-23.6966, -11.0521) (-23.7601, -10.9569) (-23.7839, -10.9807) knots 0 0 0 0 1 1 1 1
  spline S162 degree 3 poles (-23.7839, -10.9807) (-23.8553, -11.0521) (-23.3394, -12.8936) (-23.0933, -13.4254) knots 0 0 0 0 1 1 1 1
  spline S163 degree 3 poles (-23.0933, -13.4254) (-22.3393, -15.0526) (-21.4582, -14.3462) (-20.7597, -11.5601) knots 0 0 0 0 1 1 1 1
  spline S164 degree 3 poles (-20.7597, -11.5601) (-20.6486, -11.1315) (-20.5613, -10.7108) (-20.5613, -10.6314) knots 0 0 0 0 1 1 1 1
  spline S165 degree 3 poles (-20.5613, -10.6314) (-20.5613, -10.5441) (-20.5374, -10.4806) (-20.4978, -10.4806) knots 0 0 0 0 1 1 1 1
  spline S166 degree 3 poles (-20.4978, -10.4806) (-20.466, -10.4806) (-20.3628, -10.8934) (-20.2596, -11.4014) knots 0 0 0 0 1 1 1 1
  spline S167 degree 3 poles (-20.2596, -11.4014) (-19.069, -17.4101) (-15.4971, -22.5774) (-11.4093, -24.2125) knots 0 0 0 0 1 1 1 1
  spline S168 degree 3 poles (-11.4093, -24.2125) (-10.3378, -24.6411) (-9.5281, -24.7919) (-8.3772, -24.7919) knots 0 0 0 0 1 1 1 1
  spline S169 degree 3 poles (-8.3772, -24.7919) (-7.1707, -24.784) (-6.6389, -24.6649) (-7.4723, -24.5856) knots 0 0 0 0 1 1 1 1
  spline S170 degree 3 poles (-7.4723, -24.5856) (-9.9964, -24.3474) (-12.7825, -22.4345) (-14.8859, -19.4897) knots 0 0 0 0 1 1 1 1
  spline S171 degree 3 poles (-14.8859, -19.4897) (-15.4892, -18.6404) (-16.7513, -16.4496) (-16.7513, -16.2353) knots 0 0 0 0 1 1 1 1
  spline S172 degree 3 poles (-16.7513, -16.2353) (-16.7513, -16.2036) (-16.5211, -16.5211) (-16.2353, -16.9497) knots 0 0 0 0 1 1 1 1
  spline S173 degree 3 poles (-16.2353, -16.9497) (-14.3065, -19.831) (-11.4887, -22.2916) (-8.4566, -23.7442) knots 0 0 0 0 1 1 1 1
  spline S174 degree 3 poles (-8.4566, -23.7442) (-6.0277, -24.9031) (-3.7655, -25.4031) (-1.3525, -25.292) knots 0 0 0 0 1 1 1 1
  spline S175 degree 3 poles (-1.3525, -25.292) (0.4414, -25.2206) (1.8542, -24.8634) (3.2751, -24.1411) knots 0 0 0 0 1 1 1 1
  spline S176 degree 3 poles (3.2751, -24.1411) (3.9656, -23.7839) (5.3547, -22.879) (5.2912, -22.8155) knots 0 0 0 0 1 1 1 1
  spline S177 degree 3 poles (5.2912, -22.8155) (5.2753, -22.7996) (4.9975, -22.879) (4.6641, -22.9822) knots 0 0 0 0 1 1 1 1
  spline S178 degree 3 poles (4.6641, -22.9822) (3.283, -23.4187) (2.5289, -23.5299) (0.8303, -23.5299) knots 0 0 0 0 1 1 1 1
  spline S179 degree 3 poles (0.8303, -23.5299) (-1.1223, -23.5378) (-2.1145, -23.3791) (-4.0116, -22.7679) knots 0 0 0 0 1 1 1 1
  line L33 (-4.0116, -22.7679) -> (-4.8053, -22.5059)
  line L34 (-4.8053, -22.5059) -> (-3.7734, -22.4583)
  spline S180 degree 3 poles (-3.7734, -22.4583) (-2.7416, -22.4107) (-2.1145, -22.2916) (-1.2493, -21.9741) knots 0 0 0 0 1 1 1 1
  spline S181 degree 3 poles (-1.2493, -21.9741) (-1.0033, -21.8868) (-0.7969, -21.8074) (-0.7969, -21.7995) knots 0 0 0 0 1 1 1 1
  spline S182 degree 3 poles (-0.7969, -21.7995) (-0.7969, -21.7916) (-1.2573, -21.7995) (-1.8288, -21.8154) knots 0 0 0 0 1 1 1 1
  spline S183 degree 3 poles (-1.8288, -21.8154) (-3.0829, -21.8551) (-3.8925, -21.7439) (-4.9958, -21.3867) knots 0 0 0 0 1 1 1 1
  spline S184 degree 3 poles (-4.9958, -21.3867) (-9.7266, -19.8389) (-14.116, -14.8701) (-16.275, -8.6153) knots 0 0 0 0 1 1 1 1
  spline S185 degree 3 poles (-16.275, -8.6153) (-16.6401, -7.5517) (-17.0132, -6.2182) (-16.9735, -6.115) knots 0 0 0 0 1 1 1 1
  spline S186 degree 3 poles (-16.9735, -6.115) (-16.9576, -6.0753) (-16.6957, -6.2023) (-16.3941, -6.4007) knots 0 0 0 0 1 1 1 1
  spline S187 degree 3 poles (-16.3941, -6.4007) (-15.5289, -6.9643) (-13.3937, -7.9803) (-12.338, -8.3296) knots 0 0 0 0 1 1 1 1
  spline S188 degree 3 poles (-12.338, -8.3296) (-10.6711, -8.8852) (-9.9329, -9.0043) (-8.2581, -9.0122) knots 0 0 0 0 1 1 1 1
  spline S189 degree 3 poles (-8.2581, -9.0122) (-6.9643, -9.0122) (-6.7183, -8.9884) (-6.1706, -8.8296) knots 0 0 0 0 1 1 1 1
  spline S190 degree 3 poles (-6.1706, -8.8296) (-5.1784, -8.5439) (-4.5513, -8.2026) (-3.9719, -7.6231) knots 0 0 0 0 1 1 1 1
  spline S191 degree 3 poles (-3.9719, -7.6231) (-3.0749, -6.7341) (-2.7257, -5.7658) (-2.813, -4.3688) knots 0 0 0 0 1 1 1 1
  spline S192 degree 3 poles (-2.813, -4.3688) (-2.8368, -3.9084) (-2.8765, -3.448) (-2.9082, -3.3369) knots 0 0 0 0 1 1 1 1
  spline S193 degree 3 poles (-2.9082, -3.3369) (-2.9479, -3.1384) (-2.9162, -3.1146) (-2.0272, -2.7813) knots 0 0 0 0 1 1 1 1
  spline S194 degree 3 poles (-2.0272, -2.7813) (-1.2414, -2.4796) (-1.0985, -2.4003) (-1.0668, -2.2256) knots 0 0 0 0 1 1 1 1
  spline S195 degree 3 poles (-1.0668, -2.2256) (0.0683, 3.1004) (4.0371, 7.0613) (8.8948, 7.7121) knots 0 0 0 0 1 1 1 1
  line L35 (8.8948, 7.7121) -> (9.5854, 7.7994)
  line L36 (9.5854, 7.7994) -> (9.633, 8.1566)
  spline S196 degree 3 poles (9.633, 8.1566) (9.7124, 8.7281) (9.6727, 9.9267) (9.5695, 10.3712) knots 0 0 0 0 1 1 1 1
  spline S197 degree 3 poles (-4.845, -3.8766) (-11.9411, -6.5595) (-18.4419, -6.0912) (-20.9899, -2.7019) knots 0 0 0 0 1 1 1 1
  spline S198 degree 3 poles (-20.9899, -2.7019) (-21.1963, -2.4241) (-21.3471, -2.1859) (-21.3233, -2.1701) knots 0 0 0 0 1 1 1 1
  spline S199 degree 3 poles (-21.3233, -2.1701) (-21.3074, -2.1542) (-21.0613, -2.3209) (-20.7835, -2.5431) knots 0 0 0 0 1 1 1 1
  spline S200 degree 3 poles (-20.7835, -2.5431) (-20.1882, -3.0273) (-18.8071, -3.7179) (-17.8228, -4.0433) knots 0 0 0 0 1 1 1 1
  spline S201 degree 3 poles (-17.8228, -4.0433) (-14.6875, -5.0514) (-10.5918, -5.0831) (-6.3849, -4.1227) knots 0 0 0 0 1 1 1 1
  spline S202 degree 3 poles (-6.3849, -4.1227) (-5.8213, -3.9957) (-5.0673, -3.8052) (-4.718, -3.6941) knots 0 0 0 0 1 1 1 1
  spline S203 degree 3 poles (-4.718, -3.6941) (-4.1148, -3.5036) (-3.9084, -3.4559) (-3.9798, -3.5274) knots 0 0 0 0 1 1 1 1
  spline S204 degree 3 poles (-3.9798, -3.5274) (-3.9957, -3.5433) (-4.3846, -3.702) (-4.845, -3.8766) knots 0 0 0 0 1 1 1 1
  arc A19 (-35.8666, 49.9584) -> (-35.5399, -50.1913) centre (0, 0) ccw
  arc A20 (-35.0849, 50.1261) -> (-35.8666, 49.9584) centre (-35.2834, 49.146) ccw
  arc A21 (35.9196, 49.9203) -> (35.1381, 50.0889) centre (35.3355, 49.1086) ccw
  arc A22 (35.5399, -50.1913) -> (58.2463, -19.7388) centre (0, 0) ccw
  arc A23 (58.2463, 19.7388) -> (35.9196, 49.9203) centre (0, 0) ccw
  arc A24 (58.2463, -19.7388) -> (58.1788, -18.9422) centre (57.2992, -19.4179) ccw
  arc A25 (58.1788, 18.9422) -> (58.2463, 19.7388) centre (57.2992, 19.4179) ccw
  line L37 (-54.8646, 12.1784) -> (-53.4396, 12.1784)
  line L38 (-35.7446, 12.1784) -> (-35.7446, 13.9784)
  circle A26 centre (-35.7446, 13.9784) radius 1.5
  point P0 (42.2474, -35.4497)
  point P1 (-42.2474, -35.4497)
  point P2 (-42.2474, 35.4497)
  dimension "d330" = 4
  dimension "d381" = 2.85
  dimension "d382" = 2.85
  dimension "d387" = 2.85
  dimension "d388" = 2.85
  dimension "d452" = 123
  dimension "d453" = 1
  dimension "d454" = 1
  dimension "d455" = 1
  dimension "d456" = 1
  dimension "d458" = 19.12
  dimension "d460" = 3
  constraint horizontal L1
  constraint horizontal L2
  constraint coincident L0 L3.start
  constraint tangent L1 A4
  constraint tangent A2 A4
  constraint tangent L1 A5
  constraint tangent A3 A5
  constraint tangent L4 A6
  constraint tangent A0 A6
  constraint tangent L3 A7
  constraint tangent A1 A7
  constraint tangent A1 A8
  constraint tangent A0 A9
  constraint tangent A2 A10
  constraint tangent A3 A11
  constraint tangent A12 A18
  constraint tangent A13 A18
  constraint equal A12 A13
  constraint vertical L5
  constraint vertical L6
  constraint collinear L7 L8
  constraint concentric A13 A14
  constraint concentric A12 A15
  constraint concentric A19 A22
  constraint tangent A19 A20
  constraint tangent A8 A20
  constraint tangent A21 A22
  constraint tangent A9 A21
  constraint concentric A22 A23
  constraint tangent A12 A24
  constraint tangent A22 A24
  constraint tangent A13 A25
  constraint tangent A23 A25
  constraint horizontal L37
  constraint vertical L38
  constraint coincident A16.centre L37.start
  constraint coincident L38.end A26.centre
  constraint coincident A16 L37.end
  measures "d330" radius of A12
  measures "d381" diameter of A14
  measures "d382" diameter of A15
  measures "d387" diameter of A16
  measures "d388" diameter of A17
  measures "d452" diameter of A22
  measures "d453" radius of A20
  measures "d454" radius of A21
  measures "d455" radius of A24
  measures "d456" radius of A25
  measures "d458" distance of A16.centre L38.start
  measures "d460" diameter of A26
extrude "Extrude44" add sketch "Sketch6" along normal blind 4 contours L0 L1 L2 L3 L4 A0 A1 A2 A3 A4 A5 A6 A7 A8 A9 A10 A11 A12 A13 A18 A19 A20 A21 A22 A23 A24 A25 | A26
extrude "Extrude45" add sketch "Sketch6" along normal blind 3 contours S0 S1 L9 L10 S2 S3 S4 S5 S6 S7 S8 S9 S10 S11 L11 L12 S12 S13 S14 L13 L14 S15 S16 S17 S18 S19 S20 S21 S22 S23 S24 S25 S26 S27 S28 L15 L16 S29 S30 S31 S32 L17 L18 S33 S34 S35 S36 S37 S38 S39 S40 S41 S42 S43 S44 S45 S46 S47 S48 S49 L19 L20 S50 S51 S52 S53 S54 S55 S56 S57 S58 S59 S60 S61 S62 S63 S64 S65 L21 L22 S66 S67 S68 S69 S70 S71 S72 S73 S74 S75 S76 S77 S78 S79 S80 S81 S82 S83 S84 S85 S86 L23 L24 S87 S88 S89 S90 S91 S92 S93 S94 S95 | S116 S117 S118 S119 S120 S121 S122 S123 S124 S125 S126 S127 S128 S129 S130 S131 S132 S133 S134 S135 S136 S137 S138 S139 L27 L28 S140 S141 S142 L29 L30 S143 S144 S145 S146 S147 S148 S149 S150 S151 S152 S153 L31 L32 S154 S155 S156 S157 S158 S159 S160 S161 S162 S163 S164 S165 S166 S167 S168 S169 S170 S171 S172 S173 S174 S175 S176 S177 S178 S179 L33 L34 S180 S181 S182 S183 S184 S185 S186 S187 S188 S189 S190 S191 S192 S193 S194 S195 L35 L36 S196
extrude "Extrude46" add sketch "Sketch6" along normal blind 4 contours S96 S97 S98 S99 S100 | S101 S102 S103 S104 S105 S106 L25 L26 S107 S108 S109 S110 S111 S112 | S197 S198 S199 S200 S201 S202 S203 S204
extrude "Extrude47" add sketch "Sketch6" along normal blind 3 contours S113 S114 S115
fillet "Fillet24" radius 1 2 edges at (35.5399, 2, 50.1913) (-35.5399, 2, 50.1913)
extrude "Extrude48" cut sketch "Sketch6" along normal blind 5 contours A26
named bodies: "lid"
